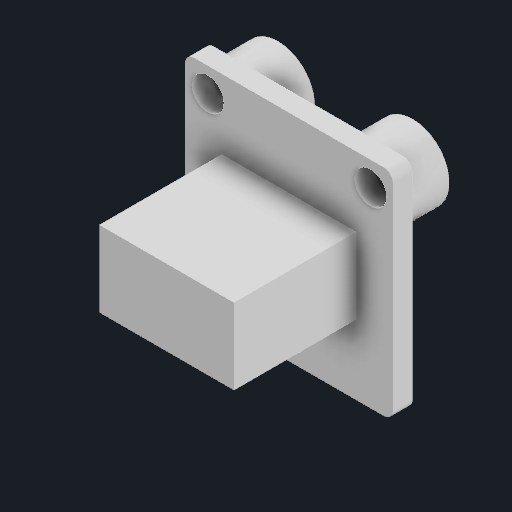
# Autodesk Inventor part: clicky pcb top
Saved by Autodesk Inventor 2024.3 (Build 283343000, 343)
## iProperties
Created: 2024-10-26
Part Number: clicky pcb top
Material: Generic
Document SubType Name: Modeling
Designer: MFil
Density: 1 g/cm^3
Appearance: Default
Author: MFil
Autodesk Inventor part; units mm, degrees
ref_plane "YZ Plane" through (0, 0, 0) normal (1, 0, 0) x (0, 1, 0)
ref_plane "XZ Plane" through (0, 0, 0) normal (0, 1, 0) x (-1, 0, 0)
ref_plane "XY Plane" through (0, 0, 0) normal (0, 0, 1) x (1, 0, 0)
sketch "Sketch1" plane through (0, 0, 0) normal (0, 0, 1) x (1, 0, 0)
  line L0 (0, 0) -> (17, 0)
  line L1 (17, 0) -> (17, 17.6)
  line L2 (17, 17.6) -> (0, 17.6)
  line L3 (0, 17.6) -> (0, 0)
  circle A0 centre (16.25, 16.85) radius 0.75
  circle A1 centre (0.75, 16.85) radius 0.75
  circle A2 centre (0.75, 0.75) radius 0.75
  circle A3 centre (16.25, 0.75) radius 0.75
  circle A4 centre (1.85, 15.6) radius 1.3
  circle A5 centre (15.15, 15.6) radius 1.3
  circle A6 centre (8.5, 2) radius 1.3
  point P0 (0, 16.85)
  point P1 (0, 0.75)
  point P2 (0.75, 0)
  point P3 (16.25, 0)
  point P4 (17, 0.75)
  point P5 (17, 16.85)
  point P6 (16.25, 17.6)
  point P7 (0.75, 17.6)
  dimension "d0" = 17
  dimension "d1" = 17.6
  dimension "d2" = 1.5
  dimension "d3" = 1.5
  dimension "d4" = 1.5
  dimension "d5" = 1.5
  dimension "d7" = 2.6
  dimension "d11" = 1.85
  dimension "d12" = 1.85
  dimension "d13" = 2
  dimension "d14" = 2.6
  dimension "d15" = 2
  dimension "d16" = 8.5
  constraints: 8 end point, 8 tangent, 7 centre point, 2 parallel, 1 equal radius, 1 horizontal, 1 horizontal alignment, 1 perpendicular
  measures "d0" distance of L2.end L1.end
  measures "d1" distance of L1.end L0.end
  measures "d2" diameter of A0
  measures "d3" diameter of A1
  measures "d4" diameter of A2
  measures "d5" diameter of A3
  measures "d7" diameter of A4
  measures "d11" distance from line of L3 A4.centre
  measures "d12" distance from line of L1 A5.centre
  measures "d13" distance from line of L2 A4.centre
  measures "d14" diameter of A6
  measures "d15" distance from line of L0 A6.centre
  measures "d16" distance from line of L1 A6.centre
extrude "Extrusion1" add sketch "Sketch1" along normal blind 1.6 contours A2 L3 A1 A4 L2 A0 A5 L1 A3 L0 | A2 | A3 | A1 A4 | A0 A5 picked at (1.0458, 16.9665) picked at (15.9541, 16.9666)
sketch "Sketch2" plane through (0, 0, 1.6) normal (0, 0, 1) x (1, 0, 0)
  line L0 (3, 11.9) -> (14, 11.9)
  line L1 (14, 11.9) -> (14, 5.7)
  line L2 (14, 5.7) -> (3, 5.7)
  line L3 (3, 5.7) -> (3, 11.9)
  line L4 (3, 11.9) -> (14, 5.7) construction
  line L5 (14, 11.9) -> (3, 5.7) construction
  line L6 (0, 16.85) -> (0, 0.75) projected
  line L7 (16.25, 17.6) -> (0.75, 17.6) projected
  point P0 (0, 0)
  point P1 (8.5, 8.8)
  point P2 (0, 8.8)
  point P3 (8.5, 17.6)
  point P4 (0, 8.8)
  point P5 (8.5, 5.7)
  dimension "d19" = 11
  dimension "d20" = 6.2
  constraints: 12 end point, 6 midpoint, 2 parallel, 1 horizontal, 1 horizontal alignment, 1 perpendicular, 1 vertical alignment
  measures "d19" distance of L0.start L0.end
  measures "d20" distance from line of point (8.5, 5.7) L0
extrude "Extrusion2" add sketch "Sketch2" along normal blind 10
sketch "Sketch3" plane through (0, 0, 0) normal (0, 0, -1) x (-1, 0, 0)
  circle A0 centre (-14, 14.6) radius 3
  circle A1 centre (-3, 14.6) radius 3
  circle A2 centre (-8.5, 3) radius 3
  circle A3 centre (-8.5, 2) radius 1.3 projected
  line L0 (-0.75, 0) -> (-16.25, 0) projected
  line L1 (-16.25, 17.6) -> (-0.75, 17.6) projected
  line L2 (-17, 0.75) -> (-17, 16.85) projected
  line L3 (0, 16.85) -> (0, 0.75) projected
  point P0 (0, 0)
  dimension "d23" = 6
  dimension "d24" = 6
  dimension "d25" = 6
  constraints: 5 tangent, 3 centre point, 1 vertical alignment
  measures "d23" diameter of A0
  measures "d24" diameter of A1
  measures "d25" diameter of A2
extrude "Extrusion3" add sketch "Sketch3" along normal blind 3 contours A0 | A1 | A2 | A3
equation "\"d12\" = d11"
body "Solid1"
